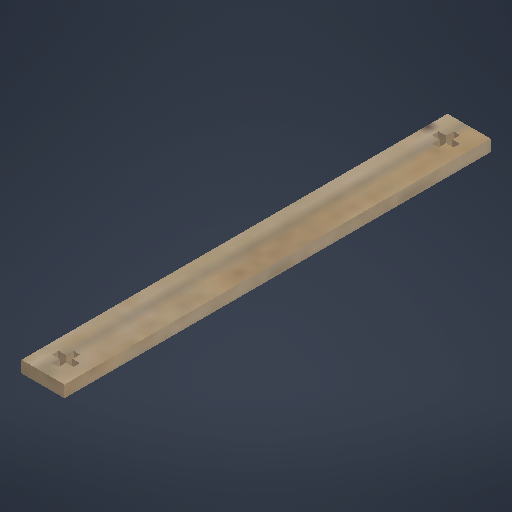
# Autodesk Inventor part: back_under
Saved by Autodesk Inventor 2026.1 (Build 301233020, 233B)
## iProperties
Created: 2025-09-28
Part Number: back_under
Material: 木材 (カエデ材)
Document SubType Name: Modeling
Designer: hibik
Density: 0.67 g/cm^3
Appearance: ナチュラル カエデ材 - 光沢 濃い着色
Author: hibik
Autodesk Inventor part; units mm, degrees
ref_plane "YZ Plane" through (0, 0, 0) normal (1, 0, 0) x (0, 1, 0)
ref_plane "XZ Plane" through (0, 0, 0) normal (0, 1, 0) x (-1, 0, 0)
ref_plane "XY Plane" through (0, 0, 0) normal (0, 0, 1) x (1, 0, 0)
sketch "スケッチ1" plane through (0, 0, 0) normal (0, 1, 0) x (-1, 0, 0)
  line L0 (0, 99) -> (20, 99)
  line L1 (20, 99) -> (20, -99)
  line L2 (20, -99) -> (0, -99)
  line L3 (0, -99) -> (0, 99)
  point P0 (0, 0)
  point P1 (0, 0)
  dimension "d0" = 198
  dimension "d1" = 20
  constraints: 8 end point, 2 parallel, 1 coincident, 1 horizontal, 1 midpoint, 1 perpendicular
  measures "d0" distance of L0.end L1.end
  measures "d1" distance of L0.start L0.end
extrude "押し出し1" add sketch "スケッチ1" along normal blind 5.5
sketch "スケッチ2" plane through (0, 5.5, 0) normal (0, 1, 0) x (1, 0, 0)
  line L0 (-15, -89.8) -> (-5, -89.8)
  line L1 (-5, -89.8) -> (-5, -86.8)
  line L2 (-5, -86.8) -> (-15, -86.8)
  line L3 (-15, -86.8) -> (-15, -89.8)
  line L4 (-8.5, -93.3) -> (-11.5, -93.3)
  line L5 (-11.5, -93.3) -> (-11.5, -83.3)
  line L6 (-11.5, -83.3) -> (-8.5, -83.3)
  line L7 (-8.5, -83.3) -> (-8.5, -93.3)
  line L8 (-20, -99) -> (0, -99) projected
  point P0 (0, 0)
  point P1 (-8.5, -88.3)
  point P2 (-15, -88.3)
  point P3 (-10, -93.3)
  point P4 (-10, -89.8)
  point P5 (-10, -99)
  point P6 (-8.5, -86.8)
  point P7 (-11.5, -86.8)
  point P8 (-11.5, -89.8)
  point P9 (-8.5, -89.8)
  point P10 (-10, -99)
  dimension "d4" = 10
  dimension "d5" = 5.7
  dimension "d6" = 3
  constraints: 16 end point, 6 midpoint, 4 parallel, 4 perpendicular, 2 horizontal, 2 vertical alignment, 1 horizontal alignment
  measures "d4" distance of L6.end L4.start
  measures "d5" distance between parallel lines of L8 L4
  measures "d6" distance of L4.start L4.end
extrude "押し出し2" cut sketch "スケッチ2" against normal through all
mirror "ミラー1" about plane through (0, 0, 0) normal (0, 0, 1) of "押し出し2"
